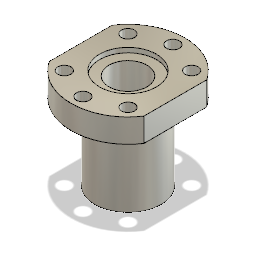
arm (Autodesk Fusion 360 archive; units mm, degrees)
design "sfu1605"
Autodesk Fusion 360 part; units mm, degrees
(part 1 of 2)
sketch "Sketch1" plane through (0, 0, 0) normal (0, 1, 0) x (1, 0, 0)
  circle A0 centre (0, 0) radius 14
  dimension "d5" = 28
  measures "d5" diameter of A0
extrude "Extrude1" add sketch "Sketch1" along normal blind 32
sketch "Sketch2" plane through (0, 32, 0) normal (0, 1, 0) x (-1, 0, 0)
  circle A0 centre (0, 0) radius 14
  line L0 (20, 13.2665) -> (20, -13.2665)
  line L1 (20, 13.2665) -> (20, -13.2665)
  line L2 (-20, 13.2665) -> (-20, -13.2665)
  arc A1 (20, 13.2665) -> (-20, 13.2665) centre (0, 0) ccw
  arc A2 (-20, -13.2665) -> (20, -13.2665) centre (0, 0) ccw
  dimension "d8" = 48
  measures "d8" diameter of A1
extrude "Extrude2" add sketch "Sketch2" along normal blind 10 contours A0 | L0 L1 L2 A1 A2
sketch "Sketch3" plane through (0, 42, 0) normal (0, 1, 0) x (-1, 0, 0)
  arc A0 (20, 13.2665) -> (-20, 13.2665) centre (0, 0) ccw
  line L0 (-20, 13.2665) -> (-20, -13.2665)
  arc A1 (-20, -13.2665) -> (20, -13.2665) centre (0, 0) ccw
  line L1 (20, -13.2665) -> (20, 13.2665)
  line L2 (20, 0) -> (10, 0)
  line L3 (-20, 0) -> (-10, 0)
  circle A2 centre (0, 0) radius 10
  dimension "d13" = 10
  dimension "d14" = 10
  measures "d14" distance of A0.centre
extrude "Extrude3" cut sketch "Sketch3" against normal through all contours A2
sketch "Sketch4" plane through (0, 42, 0) normal (0, 1, 0) x (-1, 0, 0)
  circle A0 centre (0, 0) radius 10
  arc A1 (20, 13.2665) -> (-20, 13.2665) centre (0, 0) ccw
  line L0 (-20, 13.2665) -> (-20, -13.2665)
  arc A2 (-20, -13.2665) -> (20, -13.2665) centre (0, 0) ccw
  line L1 (20, -13.2665) -> (20, 13.2665)
  circle A3 centre (0, 0) radius 12
  dimension "d16" = 24
  measures "d16" diameter of A3
extrude "Extrude4" cut sketch "Sketch4" against normal blind 2 contours A3
sketch "Sketch5" plane through (0, 42, 0) normal (0, 1, 0) x (-1, 0, 0)
  circle A0 centre (0, 0) radius 12
  arc A1 (20, 13.2665) -> (-20, 13.2665) centre (0, 0) ccw
  line L0 (-20, 13.2665) -> (-20, -13.2665)
  arc A2 (-20, -13.2665) -> (20, -13.2665) centre (0, 0) ccw
  line L1 (20, -13.2665) -> (20, 13.2665)
  circle A3 centre (0, -19) radius 2.75
  line L2 (0, 0) -> (-2, 0)
  circle A4 centre (0, 19) radius 2.75
  circle A5 centre (-13.435, -13.435) radius 2.75
  circle A6 centre (13.435, -13.435) radius 2.75
  circle A7 centre (13.435, 13.435) radius 2.75
  circle A8 centre (-13.435, 13.435) radius 2.75
  dimension "d20" = 5.5
  dimension "d29" = 5.5
  dimension "d30" = 5.5
  measures "d20" diameter of A3
  measures "d29" diameter of A5
  measures "d30" diameter of A6
extrude "Extrude5" cut sketch "Sketch5" against normal through all contours A3 | A4 | A5 | A6 | A7 | A8
sketch "Sketch6" plane through (0, 0, 0) normal (0, 1, 0) x (1, 0, 0)
  circle A0 centre (0, 0) radius 10
  circle A1 centre (0, 0) radius 8
  dimension "d32" = 20
  dimension "d33" = -2
  measures "d32" diameter of A0
extrude "Extrude6" add sketch "Sketch6" along normal blind 40

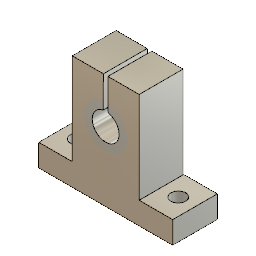
design "peca-sk8"
Autodesk Fusion 360 part; units mm, degrees
sketch "Sketch1" plane through (0, 0, 0) normal (0, 1, 0) x (1, 0, 0)
  line L0 (30, -10) -> (30, 10)
  line L1 (30, 10) -> (-30, 10)
  line L2 (-30, 10) -> (-30, -10)
  line L3 (-30, -10) -> (30, 10) construction
  line L4 (30, -10) -> (-30, 10) construction
  line L5 (-30, -10) -> (30, -10)
  line L6 (-30, -10) -> (-15, -10)
  line L7 (-15, -10) -> (15, -10)
  line L8 (15, -10) -> (15, 10)
  line L9 (15, 10) -> (-15, 10)
  line L10 (-15, 10) -> (-15, -10)
  line L11 (-15, 0) -> (-22.5, 0)
  line L12 (15, 0) -> (22.5, 0)
  dimension "d2" = 60
  dimension "d3" = 20
  dimension "d7" = 15
  dimension "d10" = 30
  dimension "d11" = 20
  dimension "d12" = 7.5
  dimension "d13" = 7.5
  measures "d12" distance of origin
  measures "d13" distance of origin
extrude "Extrude1" add sketch "Sketch1" along normal blind 10
sketch "Sketch2" plane through (0, 10, 0) normal (0, 1, 0) x (-1, 0, 0)
  line L0 (-30, -10) -> (30, -10)
  line L1 (30, -10) -> (30, 10)
  line L2 (30, 10) -> (-30, 10)
  line L3 (-30, 10) -> (-30, -10)
  line L4 (15, 10) -> (-15, 10)
  line L5 (-15, 10) -> (-15, -9.6777)
  line L6 (-15, -9.6777) -> (15, -9.6777)
  line L7 (15, -9.6777) -> (15, 10)
extrude "Extrude2" add sketch "Sketch2" along normal blind 41 contours L2 L4 L5 L6 L7
sketch "Sketch3" plane through (0, 10, 0) normal (0, 1, 0) x (-1, 0, 0)
  line L0 (-15, -9.6777) -> (-15, 10)
  line L1 (-15, 10) -> (-30, 10)
  line L2 (-30, 10) -> (-30, -10)
  line L3 (-30, -10) -> (30, -10)
  line L4 (30, -10) -> (30, 10)
  line L5 (30, 10) -> (15, 10)
  line L6 (15, 10) -> (15, -9.6777)
  line L7 (15, -9.6777) -> (-15, -9.6777)
  circle A0 centre (22.5, 0) radius 3.3
  circle A1 centre (-22.5, 0) radius 3.3
  dimension "d22" = 6.6
  dimension "d24" = 6.6
  measures "d22" diameter of A0
  measures "d24" diameter of A1
extrude "Extrude3" cut sketch "Sketch3" against normal through all contours A0 | A1
sketch "Sketch4" plane through (0, 0, 10) normal (0, 0, 1) x (1, 0, 0)
  line L0 (-30, 0) -> (30, 0)
  line L1 (30, 0) -> (30, 10)
  line L2 (30, 10) -> (15, 10)
  line L3 (15, 10) -> (15, 51)
  line L4 (15, 51) -> (-15, 51)
  line L5 (-15, 51) -> (-15, 10)
  line L6 (-15, 10) -> (-30, 10)
  line L7 (-30, 10) -> (-30, 0)
  circle A0 centre (0, 31) radius 10
  dimension "d27" = 20
  measures "d27" diameter of A0
extrude "Extrude4" cut sketch "Sketch4" against normal through all contours A0
sketch "Sketch5" plane through (0, 0, 10) normal (0, 0, 1) x (1, 0, 0)
  circle A0 centre (0, 31) radius 10
  line L0 (-30, 0) -> (30, 0)
  line L1 (30, 0) -> (30, 10)
  line L2 (30, 10) -> (15, 10)
  line L3 (15, 10) -> (15, 51)
  line L4 (15, 51) -> (-15, 51)
  line L5 (-15, 51) -> (-15, 10)
  line L6 (-15, 10) -> (-30, 10)
  line L7 (-30, 10) -> (-30, 0)
  line L8 (1, 39.4992) -> (1, 51)
  line L9 (-1.0773, 40.9418) -> (-1, 51)
  line L10 (-1, 51) -> (1, 51)
  line L11 (1, 39.4992) -> (-1.0773, 39.4992)
  line L12 (-1.0773, 40.9418) -> (-1.0773, 39.4992)
extrude "Extrude5" cut sketch "Sketch5" against normal through all contours A0 L4 L8 L9 L10 | A0 L8 L11 L12 picked at (-0.1543, 39.997)
sketch "Sketch6" plane through (0, 0, 10) normal (0, 0, 1) x (1, 0, 0)
  line L0 (1, 51) -> (1, 40.9499)
  arc A0 (-1.0773, 40.9418) -> (1, 40.9499) centre (0, 31) ccw
  line L1 (-1.0773, 40.9418) -> (-1, 51)
  line L2 (-1, 51) -> (-15, 51)
  line L3 (-15, 51) -> (-15, 10)
  line L4 (-15, 10) -> (-30, 10)
  line L5 (-30, 10) -> (-30, 0)
  line L6 (-30, 0) -> (30, 0)
  line L7 (30, 0) -> (30, 10)
  line L8 (30, 10) -> (15, 10)
  line L9 (15, 10) -> (15, 51)
  line L10 (15, 51) -> (1, 51)
move_face "OffsetFaces1" offset 4 1 faces at (-2.0526, 40.7871, -3.1185)

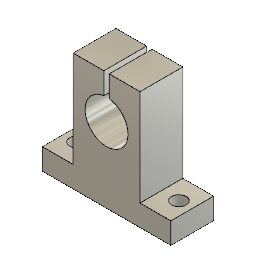
design "peca-sk8-16mm"
Autodesk Fusion 360 part; units mm, degrees
sketch "Sketch1" plane through (0, 0, 0) normal (0, 1, 0) x (1, 0, 0)
  line L0 (24, -8) -> (-24, -8)
  line L1 (-24, -8) -> (-24, 8)
  line L2 (-24, 8) -> (24, 8)
  line L3 (24, 8) -> (24, -8)
  line L4 (24, -8) -> (-24, 8) construction
  line L5 (-24, -8) -> (24, 8) construction
  line L6 (-24, -8) -> (-19, -8)
  circle A0 centre (-19, 0) radius 2.75
  circle A1 centre (19, 0) radius 2.75
  dimension "d1" = 48
  dimension "d5" = 5.5
  measures "d5" diameter of A0
extrude "Extrude1" add sketch "Sketch1" along normal blind 8
sketch "Sketch2" plane through (0, 8, 0) normal (0, 1, 0) x (-1, 0, 0)
  circle A0 centre (19, 0) radius 2.75
  circle A1 centre (-19, 0) radius 2.75
  line L0 (24, -8) -> (24, 8)
  line L1 (24, 8) -> (-24, 8)
  line L2 (-24, 8) -> (-24, -8)
  line L3 (-24, -8) -> (24, -8)
  line L4 (12.5, 8) -> (-12.5, 8)
  line L5 (-12.5, 8) -> (-12.5, -8)
  line L6 (-12.5, -8) -> (12.5, -8)
  line L7 (12.5, -8) -> (12.5, 8)
  line L8 (12.5, 8) -> (-12.5, -8) construction
  line L9 (-12.5, 8) -> (12.5, -8) construction
  dimension "d8" = 25
extrude "Extrude2" add sketch "Sketch2" along normal blind 36 contours L1 L3 L4 L5 L6 L7
sketch "Sketch3" plane through (0, 0, 8) normal (0, 0, 1) x (1, 0, 0)
  line L0 (-24, 0) -> (24, 0)
  line L1 (24, 0) -> (24, 8)
  line L2 (24, 8) -> (12.5, 8)
  line L3 (12.5, 8) -> (12.5, 44)
  line L4 (12.5, 44) -> (-12.5, 44)
  line L5 (-12.5, 44) -> (-12.5, 8)
  line L6 (-12.5, 8) -> (-24, 8)
  line L7 (-24, 8) -> (-24, 0)
  line L8 (0, 0) -> (0, 28)
  circle A0 centre (0, 28) radius 8
  dimension "d11" = 28
  dimension "d12" = 16
  measures "d12" diameter of A0
extrude "Extrude3" cut sketch "Sketch3" against normal through all contours A0
sketch "Sketch4" plane through (0, 0, 8) normal (0, 0, 1) x (1, 0, 0)
  circle A0 centre (0, 28) radius 8
  line L0 (-24, 0) -> (24, 0)
  line L1 (24, 0) -> (24, 8)
  line L2 (24, 8) -> (12.5, 8)
  line L3 (12.5, 8) -> (12.5, 44)
  line L4 (12.5, 44) -> (-12.5, 44)
  line L5 (-12.5, 44) -> (-12.5, 8)
  line L6 (-12.5, 8) -> (-24, 8)
  line L7 (-24, 8) -> (-24, 0)
  line L8 (-1, 46) -> (1, 46)
  line L9 (1, 46) -> (1, 10)
  line L10 (1, 10) -> (-1, 10)
  line L11 (-1, 10) -> (-1, 46)
  line L12 (-1, 46) -> (1, 10) construction
  line L13 (1, 46) -> (-1, 10) construction
  dimension "d14" = 2
extrude "Extrude4" cut sketch "Sketch4" against normal through all contours A0 L4 L9 L11

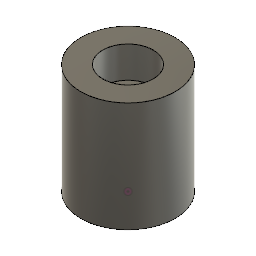
design "acoplador"
Autodesk Fusion 360 part; units mm, degrees
sketch "Sketch1" plane through (0, 0, 0) normal (0, 1, 0) x (1, 0, 0)
sketch "Sketch2" plane through (0, 0, 0) normal (0, 1, 0) x (1, 0, 0)
  circle A0 centre (0, 0) radius 15
  dimension "d2" = 30
  measures "d2" diameter of A0
extrude "Extrude1" add sketch "Sketch2" along normal blind 35
sketch "Sketch3" plane through (0, 35, 0) normal (0, 1, 0) x (-1, 0, 0)
  circle A0 centre (0, 0) radius 15
  circle A1 centre (0, 0) radius 8
  dimension "d5" = 16
  measures "d5" diameter of A1
extrude "Extrude2" cut sketch "Sketch3" against normal blind 10 contours A1
sketch "Sketch4" plane through (0, 0, 0) normal (0, 1, 0) x (1, 0, 0)
  circle A0 centre (0, 0) radius 2.5
  dimension "d8" = 5
  measures "d8" diameter of A0
extrude "Extrude3" cut sketch "Sketch4" along normal blind 8

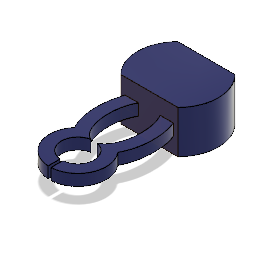
design "end-effector"
Autodesk Fusion 360 part; units mm, degrees
sketch "Sketch1" plane through (0, 0, 0) normal (0, 1, 0) x (1, 0, 0)
sketch "Sketch2" plane through (0, 0, 0) normal (0, 0, 1) x (1, 0, 0)
  line L0 (-35, -35) -> (35, -35)
  line L1 (35, -35) -> (35, 35)
  line L2 (35, 35) -> (-35, 35)
  line L3 (-35, 35) -> (-35, -35)
  line L4 (-35, -35) -> (35, 35) construction
  line L5 (35, -35) -> (-35, 35) construction
  line L6 (-35, -25.0216) -> (-70.8706, -25.0216)
  line L7 (-70.8706, -25.0216) -> (-70.8706, 52.3247)
  line L8 (-70.8706, 52.3247) -> (-35, 52.3247)
  line L9 (-35, 52.3247) -> (-35, -25.0216)
  dimension "d1" = 70
  dimension "d2" = 70
sketch "Sketch3" plane through (0, 35, 0) normal (0, 1, 0) x (-1, 0, 0)
sketch "Sketch4" plane through (0, 0, 0) normal (0, 1, 0) x (1, 0, 0)
  line L0 (-20, -20) -> (20, -20)
  line L1 (20, 20) -> (-20, 20)
  line L2 (-20, -20) -> (20, 20) construction
  line L3 (20, -20) -> (-20, 20) construction
  arc A0 (-20, 20) -> (-20, -20) centre (0, 0) ccw
  arc A1 (20, -20) -> (20, 20) centre (0, 0) ccw
  dimension "d5" = 40
extrude "Extrude2" add sketch "Sketch4" along normal blind 30
sketch "Sketch5" plane through (0, 0, 20) normal (0, 0, 1) x (1, 0, 0)
  line L0 (-20, 0) -> (20, 0)
  line L1 (20, 0) -> (20, 30)
  line L2 (20, 30) -> (-20, 30)
  line L3 (-20, 30) -> (-20, 0)
  line L4 (-28, 11) -> (28, 11)
  line L5 (28, 11) -> (28, 19)
  line L6 (28, 19) -> (-28, 19)
  line L7 (-28, 19) -> (-28, 11)
  line L8 (-28, 11) -> (28, 19) construction
  line L9 (28, 11) -> (-28, 19) construction
  dimension "d9" = 8
extrude "Extrude3" add sketch "Sketch5" along normal blind 77 contours L1 L3 L4 L6
sketch "Sketch6" plane through (0, 0, 0) normal (0, 1, 0) x (1, 0, 0)
sketch "Sketch7" plane through (0, 19, 0) normal (0, 1, 0) x (-1, 0, 0)
  line L0 (-20, 20) -> (20, 20)
  line L1 (20, 20) -> (20, 97)
  line L2 (20, 97) -> (-20, 97)
  line L3 (-20, 97) -> (-20, 20)
  line L4 (-1.798, 0) -> (0, 0)
  ellipse E0 centre (0, 36.8401) end of major axis (0, 14.5803) minor radius 11.5424 (7.5483, 20) -> (2.0744, 58.7374) ccw
  ellipse E1 centre (0, 36.8401) end of major axis (0, 14.5803) minor radius 11.5424 (-2.0744, 58.7374) -> (-7.5483, 20) ccw
  arc A0 (2.0744, 58.7374) -> (-2.0744, 58.7374) centre (0, 70) ccw
  arc A1 (15.1755, 57.2308) -> (-15.1755, 57.2308) centre (0, 70) ccw
  spline S0 degree 3 poles (16.8751, 20) (18.0673, 22.9363) (18.8803, 26.1102) (19.3749, 29.4032) (20.4602, 36.6308) (19.952, 44.3924) (17.7957, 51.1131) (17.1045, 53.2674) (16.2424, 55.3189) (15.1755, 57.2308) knots 0.908004 0.908004 0.908004 0.908004 1.288897 1.288897 1.288897 2.124892 2.124892 2.124892 2.392874 2.392874 2.392874 2.392874
  spline S1 degree 3 poles (-15.1755, 57.2308) (-15.916, 55.9038) (-16.5566, 54.5105) (-17.1114, 53.0615) (-19.3406, 47.2406) (-20.2196, 40.4918) (-19.8385, 33.8927) (-19.557, 29.0181) (-18.5925, 24.2541) (-16.8682, 20) knots -2.392874 -2.392874 -2.392874 -2.392874 -2.206922 -2.206922 -2.206922 -1.459868 -1.459868 -1.459868 -0.908051 -0.908051 -0.908051 -0.908051
  line L5 (2.0744, 58.7374) -> (-2.0744, 58.7374)
  line L6 (-1, 91) -> (-1, 80)
  line L7 (1, 91) -> (1, 80)
extrude "Extrude4" cut sketch "Sketch7" against normal through all contours L0 L1 L2 L3 A1 S0 S1 | L0 E0 E1 L5 | A0 L5 | A0 A1 L6 L7
sketch "Sketch8" plane through (0, 0, 20) normal (0, 0, 1) x (1, 0, 0)
  line L0 (-7.5483, 11) -> (-16.8751, 11)
  line L1 (-16.8751, 11) -> (-16.8751, 19)
  line L2 (-16.8751, 19) -> (-7.5483, 19)
  line L3 (-7.5483, 19) -> (-7.5483, 11)
  line L4 (-20, 30) -> (-20, 0)
  line L5 (-20, 0) -> (20, 0)
  line L6 (20, 0) -> (20, 30)
  line L7 (20, 30) -> (-20, 30)
  line L8 (7.5483, 11) -> (7.5483, 19)
  line L9 (7.5483, 19) -> (16.8682, 19)
  line L10 (16.8682, 19) -> (16.8682, 11)
  line L11 (16.8682, 11) -> (7.5483, 11)

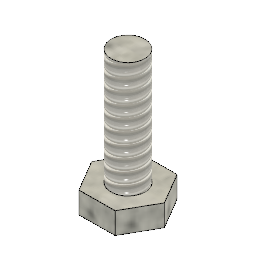
design "parafusos"
Autodesk Fusion 360 part; units mm, degrees
sketch "Sketch1" plane through (0, 0, 0) normal (0, 1, 0) x (1, 0, 0)
  circle A0 centre (0, 0) radius 2.5
  dimension "d1" = 5
  measures "d1" diameter of A0
sketch "Sketch2" plane through (0, 1, 0) normal (0, 1, 0) x (-1, 0, 0)
  circle A0 centre (0, 0) radius 2.5
  circle A1 centre (0, 0) radius 1.25
  dimension "d4" = 2.5
  measures "d4" diameter of A1
sketch "Sketch3" plane through (0, 0, 0) normal (0, -1, 0) x (1, 0, 0)
sketch "Sketch4" plane through (0, 0, 0) normal (0, 1, 0) x (1, 0, 0)
  line L0 (-1.502, -5.5747) -> (4.0768, -4.0881)
  line L1 (4.0768, -4.0881) -> (5.5788, 1.4866)
  line L2 (5.5788, 1.4866) -> (1.502, 5.5747)
  line L3 (1.502, 5.5747) -> (-4.0768, 4.0881)
  line L4 (-4.0768, 4.0881) -> (-5.5788, -1.4866)
  line L5 (-5.5788, -1.4866) -> (-1.502, -5.5747)
  dimension "d7" = 5
  measures "d7" distance of origin L5
sketch "Sketch5" plane through (0, 3, 0) normal (0, 1, 0) x (-1, 0, 0)
sketch "Sketch6" plane through (0, 0, 0) normal (0, 1, 0) x (1, 0, 0)
  line L0 (-2.4663, -4.3494) -> (2.5336, -4.3106)
  line L1 (2.5336, -4.3106) -> (4.9998, 0.0388)
  line L2 (4.9998, 0.0388) -> (2.4663, 4.3494)
  line L3 (2.4663, 4.3494) -> (-2.5336, 4.3106)
  line L4 (-2.5336, 4.3106) -> (-4.9998, -0.0388)
  line L5 (-4.9998, -0.0388) -> (-2.4663, -4.3494)
  dimension "d10" = 5
  measures "d10" distance of origin
extrude "Extrude4" add sketch "Sketch6" along normal blind 3
sketch "Sketch7" plane through (0, 3, 0) normal (0, 1, 0) x (-1, 0, 0)
  line L0 (4.9998, 0.0388) -> (2.4663, 4.3494)
  line L1 (2.4663, 4.3494) -> (-2.5336, 4.3106)
  line L2 (-2.5336, 4.3106) -> (-4.9998, -0.0388)
  line L3 (-4.9998, -0.0388) -> (-2.4663, -4.3494)
  line L4 (-2.4663, -4.3494) -> (2.5336, -4.3106)
  line L5 (2.5336, -4.3106) -> (4.9998, 0.0388)
  circle A0 centre (0, 0) radius 2.5
  dimension "d13" = 5
  measures "d13" diameter of A0
extrude "Extrude5" add sketch "Sketch7" along normal blind 16 contours A0
thread "Thread2" "Metric Forming Screw Threads 4.8 4.8x1.6 6g" major diameter 4.71 minor diameter 3.505 pitch 1.6 angle 60 resizes the face on face at (-2.4969, 13.6667, -0.1246)

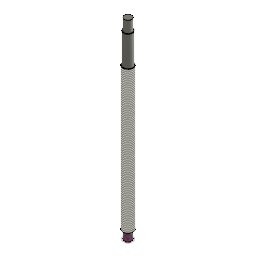
design "parafuso esfera BK/BF12"
Autodesk Fusion 360 part; units mm, degrees
sketch "Sketch1" plane through (0, 0, 0) normal (0, 1, 0) x (1, 0, 0)
sketch "Sketch2" plane through (0, 0, 0) normal (0, 1, 0) x (1, 0, 0)
  circle A0 centre (0, 0) radius 5
  dimension "d2" = 10
  measures "d2" diameter of A0
sketch "Sketch3" plane through (0, 11, 0) normal (0, 1, 0) x (-1, 0, 0)
  circle A0 centre (0, 0) radius 5
  circle A1 centre (0, 0) radius 7
  dimension "d5" = 14
  measures "d5" diameter of A1
sketch "Sketch4" plane through (0, 176, 0) normal (0, 1, 0) x (-1, 0, 0)
  circle A0 centre (0, 0) radius 6.911
  circle A1 centre (0, 0) radius 6
  dimension "d8" = 12
  measures "d8" diameter of A1
sketch "Sketch5" plane through (0, 215, 0) normal (0, 1, 0) x (-1, 0, 0)
  circle A0 centre (0, 0) radius 6
  circle A1 centre (0, 0) radius 5
  dimension "d11" = 10
  measures "d11" diameter of A1
sketch "Sketch6" plane through (0, 0, 0) normal (0, 1, 0) x (1, 0, 0)
  circle A0 centre (0, 0) radius 5
  dimension "d14" = 10
  measures "d14" diameter of A0
extrude "Extrude5" add sketch "Sketch6" along normal blind 11
sketch "Sketch7" plane through (0, 11, 0) normal (0, 1, 0) x (-1, 0, 0)
  circle A0 centre (0, 0) radius 5
  circle A1 centre (0, 0) radius 7
  dimension "d17" = 14
  measures "d17" diameter of A1
extrude "Extrude6" add sketch "Sketch7" along normal blind 185 contours A0 | A1
thread "Thread2" "ISO Metric profile 14.0 M14x2 6g" major diameter 13.822 minor diameter 11.534 pitch 2 angle 60 resizes the face on face at (-6.9652, 72.6667, -0.697)
sketch "Sketch8" plane through (0, 196, 0) normal (0, 1, 0) x (-1, 0, 0)
  circle A0 centre (0, 0) radius 6.911
  circle A1 centre (0, 0) radius 6
  dimension "d20" = 12
  measures "d20" diameter of A1
extrude "Extrude7" add sketch "Sketch8" along normal blind 39 contours A1
sketch "Sketch9" plane through (0, 235, 0) normal (0, 1, 0) x (-1, 0, 0)
  circle A0 centre (0, 0) radius 6
  circle A1 centre (0, 0) radius 5
  dimension "d23" = 10
  measures "d23" diameter of A1
extrude "Extrude8" add sketch "Sketch9" along normal blind 15 contours A1

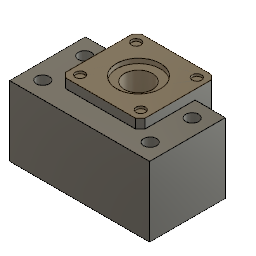
design "ballscrew-bk12"
Autodesk Fusion 360 part; units mm, degrees
sketch "Sketch1" plane through (0, 0, 0) normal (0, 1, 0) x (1, 0, 0)
  line L0 (30, 16.25) -> (-30, 16.25)
  line L1 (-30, 16.25) -> (-30, -16.25)
  line L2 (-30, -16.25) -> (30, -16.25)
  line L3 (30, -16.25) -> (30, 16.25)
  line L4 (30, 16.25) -> (-30, -16.25) construction
  line L5 (-30, 16.25) -> (30, -16.25) construction
  circle A0 centre (-23, -9) radius 2.75
  circle A1 centre (23, -9) radius 2.75
  circle A2 centre (-23, 9) radius 2.75
  circle A3 centre (23, 9) radius 2.75
  dimension "d1" = 32.5
  dimension "d2" = 60
  dimension "d6" = 5.5
  measures "d6" diameter of A0
extrude "Extrude1" add sketch "Sketch1" along normal blind 30
sketch "Sketch2" plane through (0, 30, 0) normal (0, 1, 0) x (-1, 0, 0)
  circle A0 centre (-23, 9) radius 2.75
  circle A1 centre (-23, -9) radius 2.75
  circle A2 centre (23, -9) radius 2.75
  circle A3 centre (23, 9) radius 2.75
  line L0 (-30, 16.25) -> (-30, -16.25)
  line L1 (-30, -16.25) -> (30, -16.25)
  line L2 (30, -16.25) -> (30, 16.25)
  line L3 (30, 16.25) -> (-30, 16.25)
  line L4 (17, -25.25) -> (-17, -25.25)
  line L5 (-17, -25.25) -> (-17, 7.25)
  line L6 (-17, 7.25) -> (17, 7.25)
  line L7 (17, 7.25) -> (17, -25.25)
  line L8 (17, -25.25) -> (-17, 7.25) construction
  line L9 (-17, -25.25) -> (17, 7.25) construction
  circle A4 centre (0, -9) radius 6
  dimension "d11" = 34
  dimension "d12" = 32.5
  dimension "d13" = 12
  measures "d13" diameter of A4
extrude "Extrude2" add sketch "Sketch2" along normal blind 4 contours L1 L5 L6 L7 | L1 L4 L5 L7
sketch "Sketch3" plane through (0, 34, 0) normal (0, 1, 0) x (-1, 0, 0)
  circle A0 centre (0, -9) radius 6
  line L0 (17, 7.25) -> (-17, 7.25)
  line L1 (-17, 7.25) -> (-17, -25.25)
  line L2 (-17, -25.25) -> (17, -25.25)
  line L3 (17, -25.25) -> (17, 7.25)
extrude "Extrude3" cut sketch "Sketch3" against normal through all contours A0
move_face "OffsetFaces1" offset 30 1 faces at (5.6667, 30, -19.25)
sketch "Sketch4" plane through (0, 34, 0) normal (0, 1, 0) x (-1, 0, 0)
  circle A0 centre (0, -9) radius 6
  line L0 (17, 7.25) -> (-17, 7.25)
  line L1 (-17, 7.25) -> (-17, -25.25)
  line L2 (-17, -25.25) -> (17, -25.25)
  line L3 (17, -25.25) -> (17, 7.25)
  circle A1 centre (0, -9) radius 9.3996
extrude "Extrude4" cut sketch "Sketch4" against normal blind 2 contours A1
sketch "Sketch5" plane through (0, 34, 0) normal (0, 1, 0) x (-1, 0, 0)
  circle A0 centre (0, -9) radius 9.3996
  line L0 (17, 7.25) -> (-17, 7.25)
  line L1 (-17, 7.25) -> (-17, -25.25)
  line L2 (-17, -25.25) -> (17, -25.25)
  line L3 (17, -25.25) -> (17, 7.25)
  line L4 (-17, -9) -> (17, -9)
  line L5 (0, -25.25) -> (0, 7.25)
  circle A1 centre (13, -21) radius 2
  circle A2 centre (13, -21) radius 3
  circle A3 centre (13, 3) radius 2
  circle A4 centre (13, 3) radius 3
  circle A5 centre (-13, 3) radius 3
  circle A6 centre (-13, 3) radius 2
  circle A7 centre (-13, -21) radius 2
  circle A8 centre (-13, -21) radius 3
  dimension "d23" = 1
chamfer "Chamfer1" distance 2 angle 45 4 edges at (17, 32, 7.25) (17, 17, -25.25) (-17, 17, -25.25) (-17, 32, 7.25)
extrude "Extrude5" cut sketch "Sketch5" against normal blind 1 contours A1 | A3 | A6 | A7
sketch "Sketch6" plane through (0, 34, 0) normal (0, 1, 0) x (-1, 0, 0)
  circle A0 centre (-13, 3) radius 2
  circle A1 centre (13, 3) radius 2
  circle A2 centre (-13, -21) radius 2
  circle A3 centre (13, -21) radius 2
  circle A4 centre (0, -9) radius 9.3996
  line L0 (17, 5.25) -> (15, 7.25)
  line L1 (15, 7.25) -> (-15, 7.25)
  line L2 (-15, 7.25) -> (-17, 5.25)
  line L3 (-17, 5.25) -> (-17, -23.25)
  line L4 (-17, -23.25) -> (-15, -25.25)
  line L5 (-15, -25.25) -> (15, -25.25)
  line L6 (15, -25.25) -> (17, -23.25)
  line L7 (17, -23.25) -> (17, 5.25)

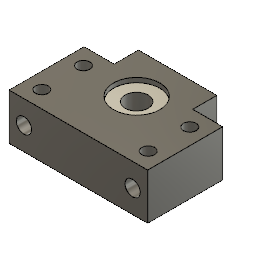
design "ballscrew-bf12"
Autodesk Fusion 360 part; units mm, degrees
sketch "Sketch1" plane through (0, 0, 0) normal (0, 1, 0) x (1, 0, 0)
  line L0 (30, -16.25) -> (-30, -16.25)
  line L1 (-30, -16.25) -> (-30, 16.25)
  line L2 (-30, 16.25) -> (30, 16.25)
  line L3 (30, 16.25) -> (30, -16.25)
  line L4 (30, -16.25) -> (-30, 16.25) construction
  line L5 (-30, -16.25) -> (30, 16.25) construction
  line L6 (0, -16.25) -> (0, 16.25)
  line L7 (-30, 0) -> (30, 0)
  line L8 (-30, -16.25) -> (-23, -16.25)
  line L9 (-30, -16.25) -> (-30, -9)
  circle A0 centre (-23, -9) radius 2.75
  dimension "d1" = 60
  dimension "d2" = 32.5
  dimension "d3" = 7
  dimension "d4" = 7.25
  dimension "d5" = 5.5
  measures "d5" diameter of A0
extrude "Extrude1" add sketch "Sketch1" along normal blind 20
sketch "Sketch2" plane through (0, 20, 0) normal (0, 1, 0) x (-1, 0, 0)
  circle A0 centre (23, 9) radius 2.75
  line L0 (30, 16.25) -> (-30, 16.25)
  line L1 (-30, 16.25) -> (-30, -16.25)
  line L2 (-30, -16.25) -> (30, -16.25)
  line L3 (30, -16.25) -> (30, 16.25)
  line L4 (30, 0) -> (-30, 0)
  line L5 (0, -16.25) -> (0, 16.25)
  circle A1 centre (-23, 9) radius 2.75
  circle A2 centre (23, -9) radius 2.75
  circle A3 centre (-23, -9) radius 2.75
extrude "Extrude2" cut sketch "Sketch2" against normal through all contours A1 | A2 | A3
sketch "Sketch3" plane through (0, 20, 0) normal (0, 1, 0) x (-1, 0, 0)
  circle A0 centre (-23, 9) radius 2.75
  circle A1 centre (-23, -9) radius 2.75
  circle A2 centre (23, -9) radius 2.75
  circle A3 centre (23, 9) radius 2.75
  line L0 (30, 16.25) -> (-30, 16.25)
  line L1 (-30, 16.25) -> (-30, -16.25)
  line L2 (-30, -16.25) -> (30, -16.25)
  line L3 (30, -16.25) -> (30, 16.25)
  line L4 (30, -16.25) -> (17, -16.25)
  line L5 (17, -16.25) -> (-17, -16.25)
  line L6 (-17, -16.25) -> (-17, -26.75)
  line L7 (-17, -26.75) -> (17, -26.75)
  line L8 (17, -26.75) -> (17, -16.25)
  line L9 (-17, -16.25) -> (-30, -16.25)
extrude "Extrude3" add sketch "Sketch3" against normal blind 20 contours L2 L5 L6 L7 L8
sketch "Sketch4" plane through (0, 20, 0) normal (0, 1, 0) x (-1, 0, 0)
  circle A0 centre (-23, 9) radius 2.75
  circle A1 centre (-23, -9) radius 2.75
  circle A2 centre (23, -9) radius 2.75
  circle A3 centre (23, 9) radius 2.75
  line L0 (30, 16.25) -> (-30, 16.25)
  line L1 (-30, 16.25) -> (-30, -16.25)
  line L2 (-30, -16.25) -> (-17, -16.25)
  line L3 (-17, -16.25) -> (-17, -26.75)
  line L4 (-17, -26.75) -> (17, -26.75)
  line L5 (17, -26.75) -> (17, -16.25)
  line L6 (17, -16.25) -> (30, -16.25)
  line L7 (30, -16.25) -> (30, 16.25)
  line L8 (0, 16.25) -> (0, -26.75)
  line L9 (23, -9) -> (-23, -9)
  circle A4 centre (0, -9) radius 5
  dimension "d14" = 10
  measures "d14" diameter of A4
extrude "Extrude4" cut sketch "Sketch4" against normal through all contours L8 L9 A4 | L8 L9 A4 | L8 L9 A4 | L8 L9 A4
sketch "Sketch5" plane through (0, 20, 0) normal (0, 1, 0) x (-1, 0, 0)
  circle A0 centre (0, -9) radius 5
  circle A1 centre (-23, 9) radius 2.75
  circle A2 centre (-23, -9) radius 2.75
  circle A3 centre (23, -9) radius 2.75
  circle A4 centre (23, 9) radius 2.75
  line L0 (30, 16.25) -> (-30, 16.25)
  line L1 (-30, 16.25) -> (-30, -16.25)
  line L2 (-30, -16.25) -> (-17, -16.25)
  line L3 (-17, -16.25) -> (-17, -26.75)
  line L4 (-17, -26.75) -> (17, -26.75)
  line L5 (17, -26.75) -> (17, -16.25)
  line L6 (17, -16.25) -> (30, -16.25)
  line L7 (30, -16.25) -> (30, 16.25)
  circle A5 centre (0, -9) radius 10
  dimension "d16" = 5
  measures "d16" distance of A0
extrude "Extrude5" cut sketch "Sketch5" against normal blind 2 contours A5
sketch "Sketch6" plane through (0, 0, -16.25) normal (0, 0, -1) x (-1, 0, 0)
  line L0 (17, 20) -> (17, 0)
  line L1 (17, 0) -> (30, 0)
  line L2 (30, 0) -> (30, 20)
  line L3 (30, 20) -> (17, 20)
  circle A0 centre (23.5, 10) radius 3.3
  line L4 (5, 0) -> (-5, 0)
  circle A1 centre (-23.5, 10) radius 3.3
  dimension "d19" = 6.6
  measures "d19" diameter of A0
extrude "Extrude6" cut sketch "Sketch6" against normal through all contours A0 | A1

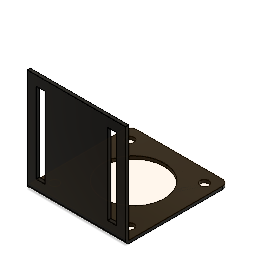
design "suporte-motor"
Autodesk Fusion 360 part; units mm, degrees
sketch "Sketch1" plane through (0, 0, 0) normal (0, 1, 0) x (1, 0, 0)
  line L0 (31, -31.5) -> (-31, -31.5)
  line L1 (-31, 31.5) -> (31, 31.5)
  line L2 (31, 31.5) -> (31, -31.5)
  line L3 (31, -31.5) -> (-31, 31.5) construction
  line L4 (-31, -31.5) -> (31, 31.5) construction
  line L5 (-31, -31.5) -> (-31, 31.5)
  circle A0 centre (0, 2.5) radius 19.25
  dimension "d2" = 62
  dimension "d4" = 38.5
  measures "d4" diameter of A0
extrude "Extrude1" add sketch "Sketch1" along normal blind 2
fillet "Fillet1" radius 4 2 edges at (31, 1, -31.5) (-31, 1, -31.5)
sketch "Sketch2" plane through (0, 2, 0) normal (0, 1, 0) x (-1, 0, 0)
  arc A0 (27, -31.5) -> (31, -27.5) centre (27, -27.5) ccw
  line L0 (31, -27.5) -> (31, 31.5)
  line L1 (31, 31.5) -> (-31, 31.5)
  line L2 (-31, 31.5) -> (-31, -27.5)
  arc A1 (-31, -27.5) -> (-27, -31.5) centre (-27, -27.5) ccw
  line L3 (-27, -31.5) -> (27, -31.5)
  circle A2 centre (0, -2.5) radius 19.25
  circle A3 centre (23.6, 23.6) radius 2.75
  circle A4 centre (23.6, -23.6) radius 2.75
  circle A5 centre (-23.6, -23.6) radius 2.75
  circle A6 centre (-23.6, 23.6) radius 2.75
  dimension "d10" = 5.5
  measures "d10" diameter of A3
extrude "Extrude2" cut sketch "Sketch2" against normal through all contours A3 | A4 | A5 | A6
sketch "Sketch3" plane through (0, 2, 0) normal (0, 1, 0) x (-1, 0, 0)
  circle A0 centre (23.6, -23.6) radius 2.75
  circle A1 centre (-23.6, -23.6) radius 2.75
  circle A2 centre (23.6, 23.6) radius 2.75
  circle A3 centre (-23.6, 23.6) radius 2.75
  arc A4 (27, -31.5) -> (31, -27.5) centre (27, -27.5) ccw
  line L0 (31, -27.5) -> (31, 31.5)
  line L1 (31, 31.5) -> (-31, 31.5)
  line L2 (-31, 31.5) -> (-31, -27.5)
  arc A5 (-31, -27.5) -> (-27, -31.5) centre (-27, -27.5) ccw
  line L3 (-27, -31.5) -> (27, -31.5)
  circle A6 centre (0, -2.5) radius 19.25
sketch "Sketch4" plane through (0, 0, 0) normal (0, -1, 0) x (1, 0, 0)
  circle A0 centre (-23.6, -23.6) radius 2.75
  circle A1 centre (23.6, -23.6) radius 2.75
  circle A2 centre (-23.6, 23.6) radius 2.75
  circle A3 centre (23.6, 23.6) radius 2.75
  circle A4 centre (0, -2.5) radius 19.25
  arc A5 (-31, -27.5) -> (-27, -31.5) centre (-27, -27.5) ccw
  line L0 (-27, -31.5) -> (27, -31.5)
  arc A6 (27, -31.5) -> (31, -27.5) centre (27, -27.5) ccw
  line L1 (31, -27.5) -> (31, 31.5)
  line L2 (31, 31.5) -> (-31, 31.5)
  line L3 (-31, 31.5) -> (-31, -27.5)
  line L4 (31, 31.5) -> (-31, 31.5)
  line L5 (-31, 31.5) -> (-31, 33.5)
  line L6 (-31, 33.5) -> (31, 33.5)
  line L7 (31, 33.5) -> (31, 31.5)
  dimension "d12" = 2
  dimension "d13" = 62
extrude "Extrude3" add sketch "Sketch4" against normal blind 65 contours L2 L4 L5 L6 L7
fillet "Fillet2" radius 2 1 edges at (0, 0, 33.5)
sketch "Sketch5" plane through (0, 0, 33.5) normal (0, 0, 1) x (1, 0, 0)
  line L0 (-31, 2) -> (31, 2)
  line L1 (31, 2) -> (31, 65)
  line L2 (31, 65) -> (-31, 65)
  line L3 (-31, 65) -> (-31, 2)
  line L4 (-31, 2) -> (-31, 33.5)
  line L5 (-19.75, 58.75) -> (-25.25, 58.75)
  line L6 (-25.25, 58.75) -> (-25.25, 8.25)
  line L7 (-25.25, 8.25) -> (-19.75, 8.25)
  line L8 (-19.75, 8.25) -> (-19.75, 58.75)
  line L9 (-19.75, 58.75) -> (-25.25, 8.25) construction
  line L10 (-25.25, 58.75) -> (-19.75, 8.25) construction
  line L11 (19.75, 8.25) -> (19.75, 58.75)
  line L12 (25.25, 58.75) -> (19.75, 8.25) construction
  line L13 (19.75, 58.75) -> (25.25, 8.25) construction
  line L14 (19.75, 58.75) -> (25.25, 58.75)
  line L15 (25.25, 8.25) -> (19.75, 8.25)
  line L16 (25.25, 58.75) -> (25.25, 8.25)
extrude "Extrude4" cut sketch "Sketch5" against normal through all contours L5 L6 L7 L8 | L11 L14 L15 L16

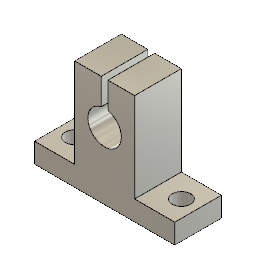
design "peca-sk8-14mm"
Autodesk Fusion 360 part; units mm, degrees
sketch "Sketch1" plane through (0, 0, 0) normal (0, 1, 0) x (1, 0, 0)
  line L0 (21, -7) -> (-21, -7)
  line L1 (-21, -7) -> (-21, 7)
  line L2 (-21, 7) -> (21, 7)
  line L3 (21, 7) -> (21, -7)
  line L4 (21, -7) -> (-21, 7) construction
  line L5 (-21, -7) -> (21, 7) construction
  line L6 (-21, -7) -> (-16, -7)
  circle A0 centre (-16, 0) radius 2.75
  line L7 (0, -7) -> (0, -6)
  circle A1 centre (16, 0) radius 2.75
  dimension "d1" = 42
  dimension "d2" = 14
  dimension "d5" = 5.5
  measures "d5" diameter of A0
extrude "Extrude1" add sketch "Sketch1" along normal blind 6
sketch "Sketch2" plane through (0, 6, 0) normal (0, 1, 0) x (-1, 0, 0)
  circle A0 centre (16, 0) radius 2.75
  circle A1 centre (-16, 0) radius 2.75
  line L0 (21, -7) -> (21, 7)
  line L1 (21, 7) -> (-21, 7)
  line L2 (-21, 7) -> (-21, -7)
  line L3 (-21, -7) -> (21, -7)
  line L4 (9, 7) -> (-9, 7)
  line L5 (-9, 7) -> (-9, -7)
  line L6 (-9, -7) -> (9, -7)
  line L7 (9, -7) -> (9, 7)
  line L8 (9, 7) -> (-9, -7) construction
  line L9 (-9, 7) -> (9, -7) construction
  dimension "d8" = 18
extrude "Extrude2" add sketch "Sketch2" along normal blind 26.8 contours L1 L3 L4 L5 L6 L7
sketch "Sketch3" plane through (0, 0, 7) normal (0, 0, 1) x (1, 0, 0)
  line L0 (-21, 0) -> (21, 0)
  line L1 (21, 0) -> (21, 6)
  line L2 (21, 6) -> (9, 6)
  line L3 (9, 6) -> (9, 32.8)
  line L4 (9, 32.8) -> (-9, 32.8)
  line L5 (-9, 32.8) -> (-9, 6)
  line L6 (-9, 6) -> (-21, 6)
  line L7 (-21, 6) -> (-21, 0)
  circle A0 centre (0, 20) radius 5
  line L8 (0, 25) -> (0, 32.8)
  dimension "d12" = 10
  measures "d12" diameter of A0
extrude "Extrude3" cut sketch "Sketch3" against normal through all contours A0
sketch "Sketch4" plane through (0, 0, 7) normal (0, 0, 1) x (1, 0, 0)
  circle A0 centre (0, 20) radius 5
  line L0 (-21, 0) -> (21, 0)
  line L1 (21, 0) -> (21, 6)
  line L2 (21, 6) -> (9, 6)
  line L3 (9, 6) -> (9, 32.8)
  line L4 (9, 32.8) -> (-9, 32.8)
  line L5 (-9, 32.8) -> (-9, 6)
  line L6 (-9, 6) -> (-21, 6)
  line L7 (-21, 6) -> (-21, 0)
  line L8 (-1, 35) -> (1, 35)
  line L9 (1, 35) -> (1, 5)
  line L10 (1, 5) -> (-1, 5)
  line L11 (-1, 5) -> (-1, 35)
  line L12 (-1, 35) -> (1, 5) construction
  line L13 (1, 35) -> (-1, 5) construction
  dimension "d16" = 30
  measures "d16" distance of origin
extrude "Extrude4" cut sketch "Sketch4" against normal through all contours A0 L4 L9 L11

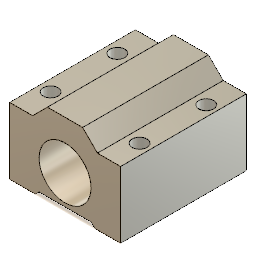
design "peca-pillow"
Autodesk Fusion 360 part; units mm, degrees
sketch "Sketch1" plane through (0, 0, 0) normal (0, 1, 0) x (1, 0, 0)
  line L0 (-15, -17) -> (15, -17)
  line L1 (15, -17) -> (15, 17)
  line L2 (15, 17) -> (-15, 17)
  line L3 (-15, 17) -> (-15, -17)
  line L4 (-15, -17) -> (15, 17) construction
  line L5 (15, -17) -> (-15, 17) construction
  dimension "d1" = 30
  dimension "d2" = 34
extrude "Extrude1" add sketch "Sketch1" along normal blind 18
sketch "Sketch2" plane through (0, 0, 17) normal (0, 0, 1) x (1, 0, 0)
  line L0 (-15, 0) -> (15, 0)
  line L1 (15, 0) -> (15, 18)
  line L2 (15, 18) -> (-15, 18)
  line L3 (-15, 18) -> (-15, 0)
  circle A0 centre (0, 9) radius 4
  dimension "d5" = 8
  measures "d5" diameter of A0
extrude "Extrude2" cut sketch "Sketch2" against normal through all contours A0
sketch "Sketch3" plane through (0, 18, 0) normal (0, 1, 0) x (-1, 0, 0)
  line L0 (-8.75, 17) -> (8.75, 17)
  line L1 (8.75, 17) -> (8.75, -17)
  line L2 (8.75, -17) -> (-8.75, -17)
  line L3 (-8.75, -17) -> (-8.75, 17)
  line L4 (-8.75, 17) -> (8.75, -17) construction
  line L5 (8.75, 17) -> (-8.75, -17) construction
  dimension "d8" = 17.5
extrude "Extrude3" add sketch "Sketch3" along normal blind 4
chamfer "Chamfer1" distance 4 angle 45 2 edges at (8.75, 22, 0) (-8.75, 22, 0)
sketch "Sketch4" plane through (0, 0, 17) normal (0, 0, 1) x (1, 0, 0)
  circle A0 centre (0, 9) radius 4
  line L0 (-4.75, 22) -> (-8.75, 18)
  line L1 (-8.75, 18) -> (-15, 18)
  line L2 (-15, 18) -> (-15, 0)
  line L3 (-15, 0) -> (15, 0)
  line L4 (15, 0) -> (15, 18)
  line L5 (15, 18) -> (8.75, 18)
  line L6 (8.75, 18) -> (4.75, 22)
  line L7 (4.75, 22) -> (-4.75, 22)
  circle A1 centre (0, 9) radius 7
extrude "Extrude4" cut sketch "Sketch4" against normal through all contours A1
sketch "Sketch5" plane through (0, 22, 0) normal (0, 1, 0) x (-1, 0, 0)
  line L0 (4.75, -17) -> (4.75, 17)
  line L1 (4.75, 17) -> (-4.75, 17)
  line L2 (-4.75, 17) -> (-4.75, -17)
  line L3 (-4.75, -17) -> (4.75, -17)
  line L4 (8.75, -17) -> (15, -17)
  line L5 (11.875, -17) -> (11.875, -9)
  circle A0 centre (11.875, -9) radius 2
  line L6 (11.875, -9) -> (11.875, 9)
  circle A1 centre (11.875, 9) radius 2
  line L7 (11.875, -9) -> (-12.125, -9)
  line L8 (11.875, 9) -> (-12.125, 9)
  circle A2 centre (-12.125, 9) radius 2
  circle A3 centre (-12.125, -9) radius 2
  dimension "d13" = 8
  dimension "d14" = 4
  dimension "d15" = 18
  dimension "d16" = 4
  dimension "d17" = 34
  dimension "d18" = 24
  dimension "d19" = 24
  dimension "d20" = 4
  dimension "d21" = 4
  measures "d14" diameter of A0
  measures "d16" diameter of A1
  measures "d20" diameter of A2
  measures "d21" diameter of A3
extrude "Extrude5" cut sketch "Sketch5" against normal through all contours L5 A0 L7 | A0 L6 L7 | L6 A1 L8 | L6 A1 L8 | L5 A0 L6 | A2 | A3
sketch "Sketch6" plane through (0, 0, 0) normal (0, -1, 0) x (1, 0, 0)
  circle A0 centre (12.125, -9) radius 2
  circle A1 centre (-11.875, -9) radius 2
  circle A2 centre (12.125, 9) radius 2
  circle A3 centre (-11.875, 9) radius 2
  line L0 (-15, 17) -> (-15, -17)
  line L1 (-15, -17) -> (15, -17)
  line L2 (15, -17) -> (15, 17)
  line L3 (15, 17) -> (-15, 17)
  line L4 (-7, 17) -> (7, 17)
  line L5 (7, 17) -> (7, -17)
  line L6 (7, -17) -> (-7, -17)
  line L7 (-7, -17) -> (-7, 17)
  line L8 (-7, 17) -> (7, -17) construction
  line L9 (7, 17) -> (-7, -17) construction
  dimension "d24" = 14
sketch "Sketch7" plane through (0, 0, 17) normal (0, 0, 1) x (1, 0, 0)
  circle A0 centre (0, 9) radius 7
  line L0 (-4.75, 22) -> (-8.75, 18)
  line L1 (-8.75, 18) -> (-15, 18)
  line L2 (-15, 18) -> (-15, 0)
  line L3 (-15, 0) -> (15, 0)
  line L4 (15, 0) -> (15, 18)
  line L5 (15, 18) -> (8.75, 18)
  line L6 (8.75, 18) -> (4.75, 22)
  line L7 (4.75, 22) -> (-4.75, 22)
  dimension "d23" = 14
  measures "d23" diameter of A0
extrude "Extrude6" cut sketch "Sketch6" against normal blind 1 contours L1 L3 L4 L5 L6 L7
chamfer "Chamfer2" distance 1 angle 45 2 edges at (7, 0, 0) (-7, 0, 0)

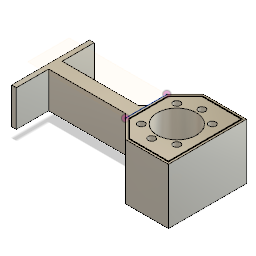
design "bracket-circular"
Autodesk Fusion 360 part; units mm, degrees
sketch "Sketch1" plane through (0, 0, 0) normal (0, 1, 0) x (1, 0, 0)
  line L0 (20, -26) -> (-20, -26)
  line L1 (-20, -26) -> (-20, 26)
  line L2 (-20, 26) -> (20, 26)
  line L3 (20, 26) -> (20, -26)
  line L4 (20, -26) -> (-20, 26) construction
  line L5 (-20, -26) -> (20, 26) construction
  dimension "d1" = 52
  dimension "d2" = 40
extrude "Extrude1" add sketch "Sketch1" along normal blind 40 makes body 1
sketch "Sketch2" plane through (0, 40, 0) normal (0, 1, 0) x (-1, 0, 0)
  line L0 (-20, -26) -> (20, -26)
  line L1 (20, -26) -> (20, 26)
  line L2 (20, 26) -> (-20, 26)
  line L3 (-20, 26) -> (-20, -26)
  circle A0 centre (0, 0) radius 14
  dimension "d5" = 28
  measures "d5" diameter of A0
extrude "Extrude2" cut sketch "Sketch2" against normal through all contours A0 bodies 1
sketch "Sketch3" plane through (0, 40, 0) normal (0, 1, 0) x (-1, 0, 0)
  circle A0 centre (0, 18) radius 2.5
  circle A1 centre (0, -18) radius 2.5
  circle A2 centre (-12.7279, -12.7279) radius 2.5
  circle A3 centre (12.7279, -12.7279) radius 2.5
  circle A4 centre (-12.7279, 12.7279) radius 2.5
  circle A5 centre (12.7279, 12.7279) radius 2.5
  dimension "d9" = 5
  dimension "d11" = 5
  dimension "d15" = 5
  dimension "d16" = 5
  dimension "d19" = 5
  dimension "d20" = 5
  measures "d9" diameter of A0
  measures "d11" diameter of A1
  measures "d15" diameter of A2
  measures "d16" diameter of A3
  measures "d19" diameter of A4
  measures "d20" diameter of A5
extrude "Extrude3" cut sketch "Sketch3" against normal blind 20 bodies 1
chamfer "Chamfer1" distance 12 angle 45 1 edges at (-20, 20, 26) on bodies 1
chamfer "Chamfer2" distance 12 angle 45 1 edges at (-20, 20, -26) on bodies 1
sketch "Sketch4" plane through (0, 40, 0) normal (0, 1, 0) x (-1, 0, 0)
  line L0 (8, -26) -> (20, -14)
  line L1 (20, -14) -> (20, 14)
  line L2 (20, 14) -> (8, 26)
  line L3 (8, 26) -> (-20, 26)
  line L4 (-20, 26) -> (-20, -26)
  line L5 (-20, -26) -> (8, -26)
  circle A0 centre (-12.7279, 12.7279) radius 2.5
  circle A1 centre (12.7279, -12.7279) radius 2.5
  circle A2 centre (0, 18) radius 2.5
  circle A3 centre (-12.7279, -12.7279) radius 2.5
  circle A4 centre (0, -18) radius 2.5
  circle A5 centre (12.7279, 12.7279) radius 2.5
  circle A6 centre (0, 0) radius 14
  line L6 (22, 14.8284) -> (8.8284, 28)
  line L7 (8.8284, 28) -> (-22, 28)
  line L8 (-22, 28) -> (-22, -28)
  line L9 (-22, -28) -> (8.8284, -28)
  line L10 (8.8284, -28) -> (22, -14.8284)
  line L11 (22, -14.8284) -> (22, 14.8284)
  line L12 (-20.6, 26.6) -> (-20.6, -26.6)
  line L13 (-20.6, -26.6) -> (8.2485, -26.6)
  line L14 (8.2485, -26.6) -> (20.6, -14.2485)
  line L15 (20.6, -14.2485) -> (20.6, 14.2485)
  line L16 (20.6, 14.2485) -> (8.2485, 26.6)
  line L17 (8.2485, 26.6) -> (-20.6, 26.6)
  dimension "d34" = 2
  dimension "d38" = 0.6
  measures "d34" distance of L2
sketch "Sketch5" plane through (20, 0, 0) normal (1, 0, 0) x (0, 0, -1)
  line L0 (-26, 0) -> (26, 0)
  line L1 (26, 0) -> (26, 40)
  line L2 (26, 40) -> (-26, 40)
  line L3 (-26, 40) -> (-26, 0)
  circle A0 centre (-20, 8) radius 2.5
  circle A1 centre (20, 8) radius 2.5
  circle A2 centre (-20, 32) radius 2.5
  circle A3 centre (20, 32) radius 2.5
  dimension "d30" = 5
  measures "d30" diameter of A0
extrude "Extrude4" cut sketch "Sketch5" against normal blind 10 contours A0 | A1 | A2 | A3 bodies 1
extrude "Extrude5" add sketch "Sketch4" against normal blind 40 separate body contours L6 L7 L8 L9 L10 L11 makes body 2
sketch "Sketch6" plane through (-22, 0, 0) normal (-1, 0, 0) x (0, 0, 1)
  line L0 (14.8284, 40) -> (-14.8284, 40)
  line L1 (-14.8284, 40) -> (-14.8284, 0)
  line L2 (-14.8284, 0) -> (14.8284, 0)
  line L3 (14.8284, 0) -> (14.8284, 40)
  line L4 (-28, 15) -> (28, 15)
  line L5 (28, 15) -> (28, 25)
  line L6 (28, 25) -> (-28, 25)
  line L7 (-28, 25) -> (-28, 15)
  line L8 (-28, 15) -> (28, 25) construction
  line L9 (28, 15) -> (-28, 25) construction
  dimension "d41" = 10
  measures "d41" distance of origin
extrude "Extrude6" add sketch "Sketch6" along normal blind 70 contours L3 L4 L5 L6 | L1 L3 L4 L6 | L1 L4 L6 L7 bodies 2
sketch "Sketch7" plane through (0, 20, 0) normal (0, 1, 0) x (-1, 0, 0)
  circle A0 centre (-12.7279, 12.7279) radius 2.5
delete_face "DeleteFace1" 1 faces at (-68.6667, 25, 4.9428) on bodies 2
extrude "Extrude7" add 1 faces at (-22, 13.3333, 4.9428) along direction (-1, 0, 0) blind 70 on bodies 2 bodies 2
sketch "Sketch8" plane through (0, 40, 0) normal (0, 1, 0) x (-1, 0, 0)
  line L0 (-20.6, 26.6) -> (8.2485, 26.6)
  line L1 (8.2485, 26.6) -> (20.6, 14.2485)
  line L2 (20.6, 14.2485) -> (20.6, -14.2485)
  line L3 (20.6, -14.2485) -> (8.2485, -26.6)
  line L4 (8.2485, -26.6) -> (-20.6, -26.6)
  line L5 (-20.6, -26.6) -> (-20.6, 26.6)
  line L6 (22, 14.8284) -> (8.8284, 28)
  line L7 (8.8284, 28) -> (-22, 28)
  line L8 (-22, 28) -> (-22, -28)
  line L9 (-22, -28) -> (8.8284, -28)
  line L10 (8.8284, -28) -> (22, -14.8284)
  line L11 (22, -14.8284) -> (92, -14.8284)
  line L12 (92, -14.8284) -> (92, 14.8284)
  line L13 (92, 14.8284) -> (22, 14.8284)
  line L14 (22, 14.8284) -> (22, -14.8284)
move_face "OffsetFaces1" offset -10 2 faces at (-45.3333, 13.3333, 14.8284) (-68.6667, 26.6667, -14.8284) on bodies 2
sketch "Sketch9" plane through (0, 40, 0) normal (0, 1, 0) x (-1, 0, 0)
  line L0 (-20.6, 26.6) -> (8.2485, 26.6)
  line L1 (8.2485, 26.6) -> (20.6, 14.2485)
  line L2 (20.6, 14.2485) -> (20.6, -14.2485)
  line L3 (20.6, -14.2485) -> (8.2485, -26.6)
  line L4 (8.2485, -26.6) -> (-20.6, -26.6)
  line L5 (-20.6, -26.6) -> (-20.6, 26.6)
  line L6 (8.8284, 28) -> (-22, 28)
  line L7 (-22, 28) -> (-22, -28)
  line L8 (-22, -28) -> (8.8284, -28)
  line L9 (8.8284, -28) -> (32, -4.8284)
  line L10 (32, -4.8284) -> (92, -4.8284)
  line L11 (92, -4.8284) -> (92, 4.8284)
  line L12 (92, 4.8284) -> (32, 4.8284)
  line L13 (22, -14.8284) -> (22, 14.8284)
  line L14 (22, 14.8284) -> (92, 14.8284)
  line L15 (92, 14.8284) -> (92, -14.8284)
  line L16 (92, -14.8284) -> (22, -14.8284)
sketch "Sketch10" plane through (0, 0, 0) normal (0, -1, 0) x (1, 0, 0)
  line L0 (-8.2485, 26.6) -> (20.6, 26.6)
  line L1 (20.6, 26.6) -> (20.6, -26.6)
  line L2 (20.6, -26.6) -> (-8.2485, -26.6)
  line L3 (-8.2485, -26.6) -> (-20.6, -14.2485)
  line L4 (-20.6, -14.2485) -> (-20.6, 14.2485)
  line L5 (-20.6, 14.2485) -> (-8.2485, 26.6)
  line L6 (-32, -4.8284) -> (-8.8284, -28)
  line L7 (-8.8284, -28) -> (22, -28)
  line L8 (22, -28) -> (22, 28)
  line L9 (22, 28) -> (-8.8284, 28)
  line L10 (-8.8284, 28) -> (-32, 4.8284)
  line L11 (-32, 4.8284) -> (-92, 4.8284)
  line L12 (-92, 4.8284) -> (-92, -4.8284)
  line L13 (-92, -4.8284) -> (-32, -4.8284)
  line L14 (-92, 14.8284) -> (-92, -14.8284)
  line L15 (-92, -14.8284) -> (-22, -14.8284)
  line L16 (-22, -14.8284) -> (-22, 14.8284)
  line L17 (-22, 14.8284) -> (-92, 14.8284)
extrude "Extrude8" cut sketch "Sketch9" against normal blind 10 contours L9 L10 L11 L13 L14 L15 | L9 L10 L15 L16 bodies 2
extrude "Extrude9" cut sketch "Sketch10" against normal blind 10 contours L6 L10 L11 L12 L13 L14 L16 | L6 L13 L14 L15 | L10 L11 L14 L17 bodies 2
sketch "Sketch11" plane through (-92, 0, 0) normal (-1, 0, 0) x (0, 0, 1)
  line L0 (-4.8284, 10) -> (4.8284, 10)
  line L1 (4.8284, 10) -> (4.8284, 30)
  line L2 (4.8284, 30) -> (-4.8284, 30)
  line L3 (-4.8284, 30) -> (-4.8284, 10)
  line L4 (-28, 10) -> (28, 10)
  line L5 (28, 10) -> (28, 30)
  line L6 (28, 30) -> (-28, 30)
  line L7 (-28, 30) -> (-28, 10)
  line L8 (-28, 10) -> (28, 30) construction
  line L9 (28, 10) -> (-28, 30) construction
extrude "Extrude10" add sketch "Sketch11" against normal blind 10 bodies 2
move_face "OffsetFaces2" offset -5 1 faces at (-92, 16.6667, -9.3333) on bodies 2
extrude "Extrude11" cut 1 faces at (-87, 16.6667, -9.3333) along direction (1, 0, 0) blind 15 on bodies 2 bodies 2
sketch "Sketch12" plane through (-72, 0, 0) normal (-1, 0, 0) x (0, 0, 1)
  line L0 (4.8284, 10) -> (4.8284, 30)
  line L1 (4.8284, 30) -> (-4.8284, 30)
  line L2 (-4.8284, 30) -> (-4.8284, 10)
  line L3 (-4.8284, 10) -> (4.8284, 10)
  line L4 (-28, 10) -> (28, 10)
  line L5 (28, 10) -> (28, 30)
  line L6 (28, 30) -> (-28, 30)
  line L7 (-28, 30) -> (-28, 10)
  line L8 (-28, 10) -> (28, 30) construction
  line L9 (28, 10) -> (-28, 30) construction
  line L10 (-28, 40) -> (-28, 0)
extrude "Extrude12" add sketch "Sketch12" along normal blind 15 contours L0 L1 L2 L3 L4 L6 bodies 2
sketch "Sketch13" plane through (-87, 0, 0) normal (-1, 0, 0) x (0, 0, 1)
  line L0 (4.8284, 10) -> (4.8284, 30)
  line L1 (4.8284, 30) -> (-4.8284, 30)
  line L2 (-4.8284, 30) -> (-4.8284, 10)
  line L3 (-4.8284, 10) -> (4.8284, 10)
  line L4 (-28, 10) -> (28, 10)
  line L5 (28, 10) -> (28, 30)
  line L6 (28, 30) -> (-28, 30)
  line L7 (-28, 30) -> (-28, 10)
  line L8 (-28, 10) -> (28, 30) construction
  line L9 (28, 10) -> (-28, 30) construction
  line L10 (-28, 40) -> (-28, 0)
extrude "Extrude13" add sketch "Sketch13" along normal blind 3.5 bodies 2
move_face "OffsetFaces3" offset 1 1 faces at (-25.3333, 10, -1.6095) on bodies 2
move_face "OffsetFaces4" offset 2 1 faces at (-25.3333, 9, -1.6095) on bodies 2
move_face "OffsetFaces5" offset 2 1 faces at (-25.3333, 30, 1.6095) on bodies 2
move_face "OffsetFaces6" offset 1 1 faces at (-25.3333, 32, 1.6095) on bodies 2

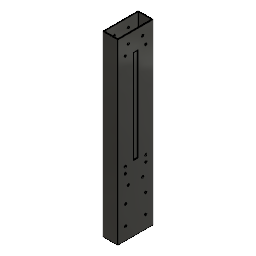
design "chapa"
Autodesk Fusion 360 part; units mm, degrees
sketch "Sketch1" plane through (0, 0, 0) normal (0, 1, 0) x (1, 0, 0)
  line L0 (-17, -40) -> (17, -40)
  line L1 (17, -40) -> (17, 40)
  line L2 (17, 40) -> (-17, 40)
  line L3 (-17, 40) -> (-17, -40)
  line L4 (-17, -40) -> (17, 40) construction
  line L5 (17, -40) -> (-17, 40) construction
  dimension "d1" = 80
  dimension "d2" = 34
extrude "Extrude1" add sketch "Sketch1" along normal blind 400
sketch "Sketch2" plane through (17, 0, 0) normal (1, 0, 0) x (0, 0, -1)
  line L0 (40, 400) -> (-40, 400)
  line L1 (-40, 400) -> (-40, 0)
  line L2 (-4.496, 357.5) -> (-4.496, 147.5)
  line L3 (-4.496, 147.5) -> (5.504, 147.5)
  line L4 (5.504, 147.5) -> (5.504, 357.5)
  line L5 (5.504, 357.5) -> (-4.496, 357.5)
  dimension "d11" = 210
  dimension "d12" = 10
extrude "Extrude2" cut sketch "Sketch2" against normal blind 34
sketch "Sketch3" plane through (0, 400, 0) normal (0, 1, 0) x (-1, 0, 0)
  line L0 (17, -40) -> (17, 40)
  line L1 (17, 40) -> (-17, 40)
  line L2 (-17, 40) -> (-17, -40)
  line L3 (-17, -40) -> (17, -40)
  line L4 (-15, 38) -> (-15, -38)
  line L5 (-15, -38) -> (15, -38)
  line L6 (15, -38) -> (15, 38)
  line L7 (15, 38) -> (-15, 38)
  dimension "d16" = 2
  measures "d16" distance of L2
extrude "Extrude3" cut sketch "Sketch3" against normal through all contours L4 L5 L6 L7
sketch "Sketch4" plane through (17, 0, 0) normal (1, 0, 0) x (0, 0, -1)
  line L0 (-4.496, 147.5) -> (-4.496, 357.5)
  line L1 (-4.496, 357.5) -> (5.504, 357.5)
  line L2 (5.504, 357.5) -> (5.504, 147.5)
  line L3 (5.504, 147.5) -> (-4.496, 147.5)
  line L4 (-40, 0) -> (40, 0)
  line L5 (40, 0) -> (40, 400)
  line L6 (40, 400) -> (-40, 400)
  line L7 (-40, 400) -> (-40, 0)
  circle A0 centre (-23, 360) radius 2.5
  circle A1 centre (23, 360) radius 2.5
  circle A2 centre (-16, 380) radius 2.5
  circle A3 centre (16, 380) radius 2.5
  dimension "d21" = 5
  dimension "d22" = 5
  dimension "d26" = 5
  dimension "d29" = 5
  measures "d21" diameter of A0
  measures "d22" diameter of A1
  measures "d26" diameter of A2
  measures "d29" diameter of A3
extrude "Extrude4" cut sketch "Sketch4" against normal through all contours A0 | A1 | A2 | A3
sketch "Sketch5" plane through (17, 0, 0) normal (1, 0, 0) x (0, 0, -1)
  circle A0 centre (-23, 360) radius 2.5
  circle A1 centre (23, 360) radius 2.5
  circle A2 centre (-16, 380) radius 2.5
  circle A3 centre (16, 380) radius 2.5
  line L0 (-4.496, 147.5) -> (-4.496, 357.5)
  line L1 (-4.496, 357.5) -> (5.504, 357.5)
  line L2 (5.504, 357.5) -> (5.504, 147.5)
  line L3 (5.504, 147.5) -> (-4.496, 147.5)
  line L4 (-40, 0) -> (40, 0)
  line L5 (40, 0) -> (40, 400)
  line L6 (40, 400) -> (-40, 400)
  circle A4 centre (-23, 145) radius 2.5
  circle A5 centre (23, 145) radius 2.5
  circle A6 centre (23, 131) radius 2.5
  circle A7 centre (-23, 131) radius 2.5
  circle A8 centre (-16, 105.5) radius 2.5
  circle A9 centre (16, 105.5) radius 2.5
  circle A10 centre (-22.5, 72) radius 2.5
  circle A11 centre (-22.5, 29) radius 2.5
  circle A12 centre (22.5, 72) radius 2.5
  circle A13 centre (22.5, 29) radius 2.5
extrude "Extrude5" cut sketch "Sketch5" against normal through all contours A4 | A5 | A6 | A7 | A8 | A9 | A10 | A11 | A12 | A13

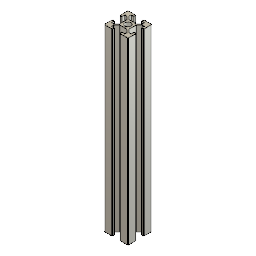
design "perfil-aluminio"
Autodesk Fusion 360 part; units mm, degrees